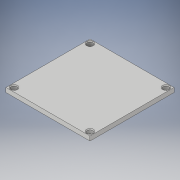
# Autodesk Inventor part: Housing_Top
Saved by Autodesk Inventor 2018 (Build 220112000, 112)
## iProperties
Created: 2018-03-28
Part Number: Housing_Top
Material: Generic
Document SubType Name: Modeling
Designer: Eric Weeks
Density: 1 g/cm^3
Appearance: Default
Author: Eric Weeks
Autodesk Inventor part; units mm, degrees
ref_plane "YZ Plane" through (0, 0, 0) normal (1, 0, 0) x (0, 1, 0)
ref_plane "XZ Plane" through (0, 0, 0) normal (0, 1, 0) x (-1, 0, 0)
ref_plane "XY Plane" through (0, 0, 0) normal (0, 0, 1) x (1, 0, 0)
sketch "Sketch1" plane through (0, 0, 0) normal (0, 1, 0) x (-1, 0, 0)
  line L0 (-15.875, -15.875) -> (15.875, -15.875)
  line L1 (15.875, -15.875) -> (15.875, 15.875)
  line L2 (15.875, 15.875) -> (-15.875, 15.875)
  line L3 (-15.875, 15.875) -> (-15.875, -15.875)
  line L4 (-15.875, -15.875) -> (15.875, 15.875) construction
  line L5 (15.875, -15.875) -> (-15.875, 15.875) construction
  point P0 (0, 0)
  point P1 (0, 0)
  dimension "d0" = 31.75
  dimension "d1" = 31.75
  constraints: 12 end point, 2 midpoint, 2 parallel, 1 coincident, 1 horizontal, 1 perpendicular
  measures "d0" distance of L2.end L1.end
  measures "d1" distance of L1.end L0.end
extrude "Extrusion1" add sketch "Sketch1" along normal blind 1.651
hole "Hole1" at (-14.351, 1.651, 14.351) direction (0, -1, 0) diameter 2.159 depth 1.651 tip angle 118 countersink diameter 2.667 countersink angle 82
hole "Hole2" at (-14.351, 1.651, -14.351) direction (0, -1, 0) diameter 2.159 depth 1.651 tip angle 118 countersink diameter 2.667 countersink angle 82
hole "Hole3" at (14.351, 1.651, -14.351) direction (0, -1, 0) diameter 2.159 depth 1.651 tip angle 118 countersink diameter 2.667 countersink angle 82
hole "Hole4" at (14.351, 1.651, 14.351) direction (0, -1, 0) diameter 2.159 depth 1.651 tip angle 118 countersink diameter 2.667 countersink angle 82
chamfer "Chamfer1" distance 0.0508 angle 45 1 edges at (-14.351, 0, 13.2715)
chamfer "Chamfer2" distance 0.0508 angle 45 1 edges at (14.351, 0, 13.2715)
chamfer "Chamfer3" distance 0.0508 angle 45 1 edges at (14.351, 0, -15.4305)
chamfer "Chamfer4" distance 0.0508 angle 45 1 edges at (-14.351, 0, -15.4305)
body "Solid1"
